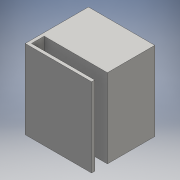
# Autodesk Inventor part: support imprimante
Saved by Autodesk Inventor 2016 (Build 200138000, 138)
## iProperties
Created: 2016-03-19
Part Number: support imprimante
Material: Generic
Document SubType Name: Modeling
Designer: Thetheos
Density: 1 g/cm^3
Appearance: Default
Author: Thetheos
Autodesk Inventor part; units mm, degrees
ref_plane "YZ Plane" through (0, 0, 0) normal (1, 0, 0) x (0, 1, 0)
ref_plane "XZ Plane" through (0, 0, 0) normal (0, 1, 0) x (-1, 0, 0)
ref_plane "XY Plane" through (0, 0, 0) normal (0, 0, 1) x (1, 0, 0)
sketch "Sketch1" plane through (0, 0, 0) normal (0, 0, 1) x (1, 0, 0)
  line L0 (0, 0) -> (42, 0)
  line L1 (42, 0) -> (42, 2)
  line L2 (42, 2) -> (2, 2)
  line L3 (2, 2) -> (2, 10)
  line L4 (2, 10) -> (42, 10)
  line L5 (42, 10) -> (42, 40)
  line L6 (42, 40) -> (0, 40)
  line L7 (0, 40) -> (0, 0)
  dimension "d0" = 42
  dimension "d1" = 40
  dimension "d2" = 30
  constraints: 16 end point, 4 perpendicular, 2 point on line, 1 horizontal
  measures "d0" distance of L0.start L0.end
  measures "d1" distance of L1.end L2.end
  measures "d2" distance of L4.end L5.end
extrude "Extrusion1" add sketch "Sketch1" along normal blind 50
body "Solid1"
